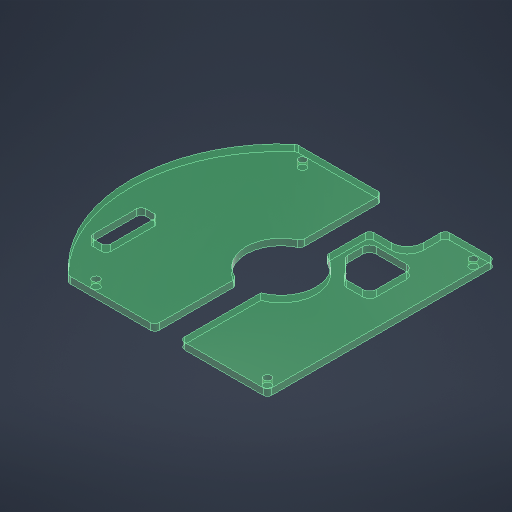
# Autodesk Inventor part: Acrilicos Superiores
Saved by Autodesk Inventor 2026.2 (Build 302298000, 298)
## iProperties
Created: 2026-02-09
Part Number: Acrilicos Superiores
Material: Generic
Document SubType Name: Modeling
Designer: 06aar
Density: 1 g/cm^3
Appearance: Clear - Green 1
Author: 06aar
Autodesk Inventor part; units mm, degrees
ref_plane "YZ Plane" through (0, 0, 0) normal (1, 0, 0) x (0, 1, 0)
ref_plane "XZ Plane" through (0, 0, 0) normal (0, 1, 0) x (-1, 0, 0)
ref_plane "XY Plane" through (0, 0, 0) normal (0, 0, 1) x (1, 0, 0)
sketch "Sketch1" plane through (0, 0, 0) normal (0, 1, 0) x (-1, 0, 0)
  line L0 (46.9204, 62.223) -> (-47, 62.223)
  line L1 (-47, -62.223) -> (46.9204, -62.223)
  line L2 (-56, 53.223) -> (-56, -53.223)
  arc A0 (50.0907, -61.0894) -> (50.0907, 61.0894) centre (0, 0) ccw
  arc A1 (50.0907, 61.0894) -> (46.9204, 62.223) centre (46.9204, 57.223) ccw
  arc A2 (46.9204, -62.223) -> (50.0907, -61.0894) centre (46.9204, -57.223) ccw
  arc A3 (-47, 62.223) -> (-56, 53.223) centre (-47, 53.223) ccw
  arc A4 (-56, -53.223) -> (-47, -62.223) centre (-47, -53.223) ccw
  line L3 (-46, 52.223) -> (45.0972, 52.223)
  arc A5 (45.0972, -52.223) -> (45.0972, 52.223) centre (0, 0) ccw
  line L4 (45.0972, -52.223) -> (-46, -52.223)
  line L5 (-46, -52.223) -> (-46, 52.223)
  circle A6 centre (0, 0) radius 8.5
  circle A7 centre (0, 0) radius 15.5
  line L6 (-5.5, -14.4914) -> (-5.5, -52.223)
  line L7 (0, 0) -> (0, -8.5)
  line L8 (5.5, -14.4914) -> (5.5, -52.223)
  line L9 (0, 0) -> (8.5, 0)
  line L10 (-5.5, 14.4914) -> (-5.5, 52.223)
  line L11 (5.5, 14.4914) -> (5.5, 52.223)
  circle A8 centre (-14.15, -43.573) radius 5.65
  line L12 (-14.15, -43.573) -> (-14.15, -52.223)
  line L13 (-5.5, -43.573) -> (-14.15, -43.573)
  line L14 (-5.5, -34.923) -> (-15.65, -34.923)
  line L15 (-22.8, -42.073) -> (-22.8, -52.223)
  arc A9 (-15.65, -34.923) -> (-22.8, -42.073) centre (-15.65, -42.073) ccw
  line L16 (45.0227, 52.023) -> (-45.8, 52.023)
  line L17 (-45.8, 52.023) -> (-45.8, -52.023)
  line L18 (-45.8, -52.023) -> (45.0227, -52.023)
  arc A10 (45.0227, -52.023) -> (45.0227, 52.023) centre (0, 0) ccw
  line L19 (5.7, -14.4914) -> (5.7, -52.223)
  circle A11 centre (0, 0) radius 16
  line L20 (5.7, 14.9503) -> (5.7, 52.223)
  line L21 (-5.7, 14.9503) -> (-5.7, 52.223)
  line L22 (-5.7, -14.4914) -> (-5.7, -52.223)
  line L23 (-23, -52.223) -> (-23, -42.073)
  arc A12 (-15.65, -34.723) -> (-23, -42.073) centre (-15.65, -42.073) ccw
  line L24 (-15.65, -34.723) -> (-5.5, -34.723)
  point P0 (48.6754, 62.223)
  point P1 (48.6754, -62.223)
  point P2 (5.5, -52.223)
  point P3 (5.5, -14.4914)
  point P4 (5.5, 14.4914)
  point P5 (5.5, 52.223)
  point P6 (-5.5, 52.223)
  point P7 (-5.5, 14.4914)
  point P8 (-22.8, -52.223)
  point P9 (-46, -32.923)
  point P10 (-23, -52.023)
  point P11 (-5.7, -34.723)
  point P12 (-5.7, -14.9503)
  point P13 (-5.7, 52.023)
  point P14 (5.7, 52.023)
  point P15 (5.7, -14.9503)
  point P16 (5.7, -52.023)
  dimension "d2" = 62.223
  dimension "d4" = 56
  dimension "d5" = 62.223
  dimension "d6" = 79
  dimension "d7" = 5
  dimension "d8" = 9
  dimension "d18" = 10
  dimension "d21" = 17
  dimension "d22" = 7
  dimension "d24" = 5.5
  dimension "d41" = 11.3
  dimension "d45" = 8.65
  dimension "d46" = 8.65
  dimension "d47" = 17.3
  dimension "d48" = 3
  dimension "d49" = 90
  dimension "d50" = 7.15
  dimension "d102" = 0.2
  dimension "d103" = 0.2
  dimension "d104" = 0.5
  dimension "d105" = 0.2
  dimension "d106" = 0.2
  dimension "d107" = 0.2
  dimension "d108" = 0.2
  constraints: 50 end point, 24 point on circle, 12 centre point, 10 tangent, 9 point on line, 7 parallel, 6 symmetric about line, 4 horizontal, 3 coincident, 2 equal radius, 2 perpendicular, 2 vertical, 11 other
  measures "d2" distance from line of point (0, 0) L0
  measures "d4" distance from line of L2 point (0, 0)
  measures "d5" distance from line of point (0, 0) L1
  measures "d6" radius of A0
  measures "d7" radius of A1
  measures "d8" radius of A3
  measures "d18" distance between parallel lines of L0 L3
  measures "d21" diameter of A6
  measures "d24" distance from line of L7.end L6
  measures "d41" diameter of A8
  measures "d45" distance of L12.start L12.end
  measures "d46" distance of L13.start L12.start
  measures "d47" distance between parallel lines of L4 L14
  measures "d48" distance edge to line of A8 L15
  measures "d49" angle of L4 L15
  measures "d50" radius of A9
  measures "d102" radial gap between concentric circles of A10 A5
  measures "d103" distance between parallel lines of L8 L19
  measures "d105" distance between parallel lines of L20 L11
  measures "d106" distance between parallel lines of L10 L21
  measures "d107" distance between parallel lines of L6 L22
  measures "d108" distance between parallel lines of L14 L24
extrude "Extrusion1" add sketch "Sketch1" against normal blind 3 contours L21 A11 L22 L24 A12 L23 L18 L17 L16 | L16 A10 L18 L19 A11 L20
fillet "Fillet11" radius 2 12 edges at (-5.7, -1.5, -14.9503) (-5.7, -1.5, 14.9503) (-5.7, -1.5, -52.023) (-45.0227, -1.5, -52.023) (5.7, -1.5, -14.9503) (5.7, -1.5, -34.723) (23, -1.5, -52.023) (45.8, -1.5, -52.023) (45.8, -1.5, 52.023) (5.7, -1.5, 52.023) (-5.7, -1.5, 52.023) (-45.0227, -1.5, 52.023)
sketch "Sketch6" plane through (0, 0, 0) normal (0, 1, 0) x (1, 0, 0)
  circle A0 centre (-37.467, 47.223) radius 1.75
  circle A1 centre (40.8, 47.023) radius 1.75
  line L0 (-7.7, 52.023) -> (-44.2712, 52.023) projected
  line L1 (-5.7, 16.2699) -> (-5.7, 50.023) projected
  line L2 (0, 0) -> (-24.1524, 0)
  circle A2 centre (-37.467, -47.223) radius 1.75
  line L3 (43.8, 52.023) -> (25, 52.023) projected
  line L4 (45.8, -50.023) -> (45.8, 50.023) projected
  circle A3 centre (40.8, -47.023) radius 1.75
  line L5 (-50, -8.023) -> (-54, -8.023)
  line L6 (-56, -10.023) -> (-56, -30.023)
  line L7 (-54, -32.023) -> (-50, -32.023)
  line L8 (-48, -30.023) -> (-48, -10.023)
  arc A4 (-48, -10.023) -> (-50, -8.023) centre (-50, -10.023) ccw
  arc A5 (-50, -32.023) -> (-48, -30.023) centre (-50, -30.023) ccw
  arc A6 (-56, -30.023) -> (-54, -32.023) centre (-54, -30.023) ccw
  arc A7 (-54, -8.023) -> (-56, -10.023) centre (-54, -10.023) ccw
  arc A8 (-45.5967, 51.5207) -> (-45.5967, -51.5207) centre (0, 0) ccw projected
  line L9 (-44.2712, -52.023) -> (-7.7, -52.023) projected
  dimension "d111" = 3.5
  dimension "d113" = 3.5
  dimension "d117" = 4.8
  dimension "d118" = 31.767
  dimension "d119" = 5
  dimension "d120" = 5
  dimension "d121" = 2
  dimension "d122" = 8
  dimension "d123" = 24
  dimension "d124" = 56
  dimension "d125" = 20
  constraints: 10 end point, 8 centre point, 8 point on circle, 8 tangent, 3 equal radius, 2 horizontal, 2 parallel, 2 symmetric about line, 1 perpendicular, 2 other
  measures "d111" diameter of A0
  measures "d113" diameter of A1
  measures "d117" distance from line of L0 A0.centre
  measures "d118" distance from line of L1 A0.centre
  measures "d119" distance from line of L3 A1.centre
  measures "d120" distance from line of L4 A1.centre
  measures "d121" radius of A4
  measures "d122" distance between parallel lines of L8 L6
  measures "d123" distance between parallel lines of L7 L5
  measures "d124" distance from line of A8.centre L6
  measures "d125" distance between parallel lines of L9 L7
extrude "Extrusion7" cut sketch "Sketch6" against normal blind 3
sketch "Sketch8" plane through (0, 0, 0) normal (0, 1, 0) x (1, 0, 0)
  line L0 (-56, -10.023) -> (-56, -30.023) projected
  arc A0 (-56, -30.023) -> (-54, -32.023) centre (-54, -30.023) ccw projected
  line L1 (-54, -32.023) -> (-50, -32.023) projected
  arc A1 (-50, -32.023) -> (-48, -30.023) centre (-50, -30.023) ccw projected
  line L2 (-48, -30.023) -> (-48, -10.023) projected
  arc A2 (-48, -10.023) -> (-50, -8.023) centre (-50, -10.023) ccw projected
  line L3 (-50, -8.023) -> (-54, -8.023) projected
  arc A3 (-54, -8.023) -> (-56, -10.023) centre (-54, -10.023) ccw projected
  circle A4 centre (-37.467, 47.223) radius 1.75 projected
  circle A5 centre (-37.467, -47.223) radius 1.75 projected
  arc A6 (-45.5967, -51.5207) -> (-44.2712, -52.023) centre (-44.2712, -50.023) ccw projected
  arc A7 (-45.5967, 51.5207) -> (-45.5967, -51.5207) centre (0, 0) ccw projected
  arc A8 (-44.2712, 52.023) -> (-45.5967, 51.5207) centre (-44.2712, 50.023) ccw projected
  line L4 (-44.2712, 52.023) -> (-7.7, 52.023) projected
  arc A9 (-5.7, 50.023) -> (-7.7, 52.023) centre (-7.7, 50.023) ccw projected
  line L5 (-5.7, 50.023) -> (-5.7, 16.2699) projected
  arc A10 (-6.8444, 14.4621) -> (-5.7, 16.2699) centre (-7.7, 16.2699) ccw projected
  arc A11 (-6.8444, 14.4621) -> (-6.8444, -14.4621) centre (0, 0) ccw projected
  arc A12 (-5.7, -16.2699) -> (-6.8444, -14.4621) centre (-7.7, -16.2699) ccw projected
  line L6 (-5.7, -16.2699) -> (-5.7, -50.023) projected
  arc A13 (-7.7, -52.023) -> (-5.7, -50.023) centre (-7.7, -50.023) ccw projected
  line L7 (-7.7, -52.023) -> (-44.2712, -52.023) projected
  circle A14 centre (40.8, 47.023) radius 1.75 projected
  circle A15 centre (40.8, -47.023) radius 1.75 projected
  arc A16 (5.7, -50.023) -> (7.7, -52.023) centre (7.7, -50.023) ccw projected
  line L8 (5.7, -50.023) -> (5.7, -14.9503) projected
  arc A17 (5.7, -14.9503) -> (6.8444, 14.4621) centre (0, 0) ccw projected
  arc A18 (5.7, 16.2699) -> (6.8444, 14.4621) centre (7.7, 16.2699) ccw projected
  line L9 (5.7, 16.2699) -> (5.7, 32.723) projected
  arc A19 (7.7, 34.723) -> (5.7, 32.723) centre (7.7, 32.723) ccw projected
  line L10 (7.7, 34.723) -> (15.65, 34.723) projected
  arc A20 (15.65, 34.723) -> (23, 42.073) centre (15.65, 42.073) ccw projected
  line L11 (23, 42.073) -> (23, 50.023) projected
  arc A21 (25, 52.023) -> (23, 50.023) centre (25, 50.023) ccw projected
  line L12 (25, 52.023) -> (43.8, 52.023) projected
  arc A22 (45.8, 50.023) -> (43.8, 52.023) centre (43.8, 50.023) ccw projected
  line L13 (45.8, 50.023) -> (45.8, -50.023) projected
  arc A23 (43.8, -52.023) -> (45.8, -50.023) centre (43.8, -50.023) ccw projected
  line L14 (43.8, -52.023) -> (7.7, -52.023) projected
  line L15 (10.7, 29.723) -> (10.7, 18.0696)
  arc A24 (10.7, -18.0696) -> (10.7, 18.0696) centre (0, 0) ccw
  line L16 (10.7, -18.0696) -> (10.7, -47.023)
  line L17 (10.7, -47.023) -> (40.8, -47.023)
  line L18 (40.8, -47.023) -> (40.8, 47.023)
  line L19 (40.8, 47.023) -> (28, 47.023)
  line L20 (28, 47.023) -> (28, 42.073)
  arc A25 (15.65, 29.723) -> (28, 42.073) centre (15.65, 42.073) ccw
  line L21 (15.65, 29.723) -> (10.7, 29.723)
  line L22 (10.7, 29.723) -> (30.7, 29.723)
  line L23 (30.7, 29.723) -> (30.7, 9.723)
  line L24 (30.7, 9.723) -> (18.6135, 9.723)
  point P0 (15.65, 29.723)
  dimension "d126" = 5
  dimension "d127" = 20
  dimension "d128" = 20
  constraints: 20 end point, 5 point on circle, 2 centre point, 2 horizontal, 1 vertical, 8 other
  measures "d126" distance between parallel lines of L9 L15
  measures "d127" distance of L22.end L23.end
  measures "d128" distance between parallel lines of L15 L23
extrude "Extrusion8" cut sketch "Sketch8" against normal blind 10 contours L22 L23 L24 A24 L15 L21
fillet "Fillet12" radius 3 5 edges at (10.7, -1.5, -29.723) (30.7, -1.5, -29.723) (10.7, -1.5, -18.0696) (18.6135, -1.5, -9.723) (30.7, -1.5, -9.723)
body "Solid1"
